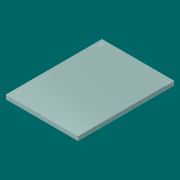
# Autodesk Inventor part: topBottom
Saved by Autodesk Inventor 2016 (Build 200138000, 138)
## iProperties
Created: 2015-10-13
Part Number: topBottom
Material: PC/ABS Plastic
Document SubType Name: Modeling
Designer: Sawaiz
Density: 0.357273 g/cm^3
Appearance: Clear
Author: Sawaiz
Autodesk Inventor part; units mm, degrees
ref_plane "YZ Plane" through (0, 0, 0) normal (1, 0, 0) x (0, 1, 0)
ref_plane "XZ Plane" through (0, 0, 0) normal (0, 1, 0) x (-1, 0, 0)
ref_plane "XY Plane" through (0, 0, 0) normal (0, 0, 1) x (1, 0, 0)
sketch "Sketch1" plane through (0, 0, 0) normal (0, 0, 1) x (1, 0, 0)
  line L0 (-76.2, -57.15) -> (76.2, -57.15)
  line L1 (76.2, -57.15) -> (76.2, 57.15)
  line L2 (76.2, 57.15) -> (-76.2, 57.15)
  line L3 (-76.2, 57.15) -> (-76.2, -57.15)
  line L4 (-76.2, -57.15) -> (76.2, 57.15) construction
  line L5 (76.2, -57.15) -> (-76.2, 57.15) construction
  point P0 (0, 0)
  dimension "d0" = 152.4
  dimension "d1" = 114.3
  constraints: 12 end point, 2 midpoint, 2 parallel, 1 horizontal, 1 perpendicular
  measures "d0" distance of L2.end L1.end
  measures "d1" distance of L1.end L0.end
extrude "Extrusion1" add sketch "Sketch1" along normal blind 6.35
sketch "Sketch10" plane through (-76.2, -57.15, 0) normal (-1, 0, 0) x (0, 0, 1)
  line L0 (0, 114.3) -> (6.35, 114.3) projected
  line L1 (3.175, 114.3) -> (3.175, 0) construction
  line L2 (0, 0) -> (6.35, 0) projected
  point P0 (0, 57.15)
  point P1 (3.175, 111.125)
  point P2 (3.175, 3.175)
  dimension "d70" = 3.175
  dimension "d71" = 3.175
  constraints: 2 end point, 2 midpoint, 2 point on line
  measures "d70" distance from line of L2 point (3.175, 3.175)
  measures "d71" distance from line of L0 point (3.175, 111.125)
hole "Hole4" at (-76.2, 53.975, 3.175) at (-76.2, -53.975, 3.175) direction (1, 0, 0) diameter 2.156 depth 8.865 tip angle 118 thread size "4-40 UNC" class "2B" standard "ANSI Unified Screw Threads"
equation "\"d0\" = depth"
equation "\"d1\" = width + 2 * acrylicThickness"
equation "\"d2\" = acrylicThickness"
equation "\"d70\" = 0.5 * acrylicThickness"
equation "\"d71\" = 0.5 * acrylicThickness"
equation "\"acrylicThickness\" = 6.35"
equation "\"width\" = 101.6"
equation "\"depth\" = 152.4"
equation "\"oRingWidth\" = 3.175"
equation "\"mirrorGroove\" = 19.05"
equation "\"mirrorGrooveMill\" = 3.175"
equation "\"height\" = 101.6"
equation "\"mirrorAngle\" = 5deg"
equation "\"detectorWidth\" = 52"
equation "\"detectorHeight\" = 52"
equation "\"mirrorThickness\" = 3.175"
equation "\"fresnelThickness\" = 0.1"
equation "\"focalLength\" = 76.2"
equation "\"ior\" = 1.49"
equation "\"centerThickness\" = 1.524"
equation "\"fresnelAngle\" = 90deg"
equation "\"fresnelEffectiveDiameter\" = 76.2"
equation "\"mirrorSuppourtWidth\" = 38.1"
equation "\"backGrooveBit\" = 4.8006"
equation "\"sensorHolderWidth\" = 88.9"
equation "\"sensorHolderHeight\" = 88.9"
equation "\"sensorHolderSensorHeight\" = 53.975"
equation "\"sensorHolderSensorWidth\" = 53.975"
equation "\"sensorHolderORingID\" = 203.2"
equation "\"sensorHolderFlushORingID\" = 304.8"
equation "\"frontBackORingID\" = 419.1"
equation "\"backMirrorGroove\" = 6.35"
equation "\"fresnelChamfer\" = 6.35"
equation "\"fresnelMirrorChamfer\" = 6.35"
equation "\"detectorOpeningHeight\" = 76.2"
equation "\"detectorOpeningWidth\" = 76.2"
body "Solid1"
